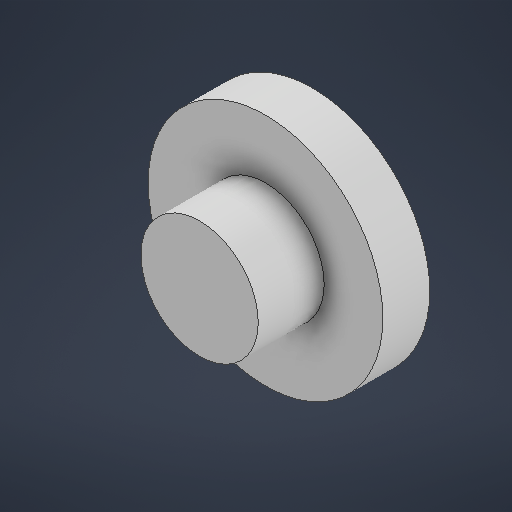
# Autodesk Inventor part: Dial
Saved by Autodesk Inventor 2026.2 (Build 302298010, 298A)
## iProperties
Created: 2026-03-03
Part Number: Dial
Material: Generic
Document SubType Name: Modeling
Designer: kjedr
Density: 1 g/cm^3
Appearance: Default
Author: kjedr
Autodesk Inventor part; units mm, degrees
ref_plane "YZ Plane" through (0, 0, 0) normal (1, 0, 0) x (0, 1, 0)
ref_plane "XZ Plane" through (0, 0, 0) normal (0, 1, 0) x (-1, 0, 0)
ref_plane "XY Plane" through (0, 0, 0) normal (0, 0, 1) x (1, 0, 0)
sketch "Sketch1" plane through (0, 0, 0) normal (0, 0, 1) x (1, 0, 0)
  circle A0 centre (0, 0) radius 22.606
  dimension "d0" = 45.212
  constraints: 1 centre point, 1 coincident
  measures "d0" diameter of A0
extrude "Extrusion1" add sketch "Sketch1" along normal blind 9.0424
sketch "Sketch2" plane through (0, 0, 9.0424) normal (0, 0, 1) x (1, 0, 0)
  circle A0 centre (0, 0) radius 11.303
  dimension "d3" = 22.606
  constraints: 1 centre point, 1 coincident
  measures "d3" diameter of A0
sketch "Sketch3" plane through (0, 0, 0) normal (0, 0, -1) x (-1, 0, 0)
  line L0 (0, -21.7935) -> (-6.35, -10.795)
  line L1 (-6.35, -10.795) -> (6.35, -10.795)
  line L2 (6.35, -10.795) -> (0, -21.7935)
  circle A0 centre (0, 0) radius 22.606 projected
  point P0 (0, -10.795)
  dimension "d4" = 12.7
  dimension "d5" = 12.7
  dimension "d7" = 60
  dimension "d8" = 10.795
  constraints: 6 end point, 1 horizontal, 1 midpoint, 1 vertical alignment
  measures "d4" distance of L0.end L1.end
  measures "d5" distance of L0.start L0.end
  measures "d7" angle of L1 L0
  measures "d8" distance of A0.centre point (0, -10.795)
extrude "Extrusion2" cut sketch "Sketch3" against normal blind 1.1303 contours L0 L1 L2
extrude "Extrusion3" add sketch "Sketch2" along normal blind 12.7
body "Solid1"
